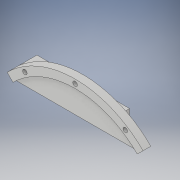
# Autodesk Inventor part: BearingGuard
Saved by Autodesk Inventor 2018 (Build 220112000, 112)
## iProperties
Created: 2019-02-07
Part Number: BearingGuard
Material: Generic
Document SubType Name: Modeling
Designer: anirudh
Density: 1 g/cm^3
Appearance: Default
Author: anirudh
Autodesk Inventor part; units mm, degrees
ref_plane "YZ Plane" through (0, 0, 0) normal (1, 0, 0) x (0, 1, 0)
ref_plane "XZ Plane" through (0, 0, 0) normal (0, 1, 0) x (-1, 0, 0)
ref_plane "XY Plane" through (0, 0, 0) normal (0, 0, 1) x (1, 0, 0)
sketch "Sketch1" plane through (0, 0, 0) normal (0, 0, 1) x (1, 0, 0)
  line L0 (0, 0) -> (101.6, 0)
  arc A0 (101.7181, 101.7181) -> (-0.1181, 101.7181) centre (50.8, 50.8) ccw
  arc A1 (106.4776, 106.4776) -> (-4.8776, 106.4776) centre (50.8, 50.8) ccw
  line L1 (0, 101.6) -> (-4.8776, 106.4776)
  line L2 (0, 101.6) -> (11.1798, 101.6) construction
  line L3 (101.6, 101.6) -> (106.4776, 106.4776)
  constraints: 8 end point, 4 point on circle, 2 centre point, 2 horizontal, 2 point on line, 1 coincident
extrude "Extrusion1" add sketch "Sketch1" along normal blind 2.54
sketch "Sketch2" plane through (0, 0, 0) normal (0, 0, -1) x (-1, 0, 0)
  line L0 (-101.7181, 101.7181) -> (0.1181, 101.7181)
  line L1 (-101.7181, 101.7181) -> (-106.4776, 106.4776) projected
  line L2 (-101.7181, 101.7181) -> (-106.4776, 106.4776)
  line L3 (4.8776, 106.4776) -> (0.1181, 101.7181) projected
  line L4 (0.1181, 101.7181) -> (4.8776, 106.4776)
  arc A0 (4.8776, 106.4776) -> (-106.4776, 106.4776) centre (-50.8, 50.8) ccw projected
  arc A1 (-106.4776, 106.4776) -> (-106.4776, 106.4776) centre (-50.8, 50.8) ccw
  point P0 (0, 0)
  constraints: 6 end point, 2 collinear, 1 horizontal, 4 other
extrude "Extrusion2" add sketch "Sketch2" along normal blind 3.81 contours L1 A0 L3 L0
sketch "Sketch8" plane through (0, 0, 2.54) normal (0, 0, 1) x (1, 0, 0)
  circle A0 centre (9.6434, 113.9463) radius 1.85
  circle A1 centre (50.8, 126.1745) radius 1.85
  circle A2 centre (91.9566, 113.9463) radius 1.85
  point P0 (0, 0)
  dimension "d32" = 3.7
  dimension "d33" = 3.7
  dimension "d34" = 3.7
  constraints: 3 centre point
  measures "d32" diameter of A0
  measures "d33" diameter of A1
  measures "d34" diameter of A2
extrude "Extrusion7" cut sketch "Sketch8" against normal blind 18.0594
sketch "Sketch9" plane through (0, 0, -3.81) normal (0, 0, -1) x (-1, 0, 0)
  line L0 (0.1181, 101.7181) -> (-71.0019, 101.7181)
  line L1 (0.1181, 101.7181) -> (4.8776, 106.4776) projected
  line L2 (0.1181, 101.7181) -> (4.8776, 106.4776)
  line L3 (4.8776, 106.4776) -> (-71.0019, 106.4776)
  line L4 (-71.0019, 106.4776) -> (-71.0019, 101.7181)
  point P0 (0, 0)
  dimension "d37" = 71.12
  constraints: 8 end point, 1 collinear, 1 horizontal
  measures "d37" distance of L0.start L0.end
extrude "Extrusion8" add sketch "Sketch9" along normal blind 18.0594
sketch "Sketch10" plane through (-4.8776, 106.4776, -3.81) normal (0, 1, 0) x (1, 0, 0)
  circle A0 centre (66.3545, 10.5594) radius 1.85
  circle A1 centre (19.05, 10.5594) radius 1.85
  circle A2 centre (42.7023, 10.5594) radius 1.85
  point P0 (4.8776, -3.81)
  point P1 (0, 18.0594)
  dimension "d44" = 3.7
  dimension "d45" = 3.7
  dimension "d46" = 3.7
  constraints: 3 centre point
  measures "d44" diameter of A0
  measures "d45" diameter of A1
  measures "d46" diameter of A2
extrude "Extrusion9" cut sketch "Sketch10" against normal blind 18.0594
fillet "Fillet3" radius 6.35 1 edges at (33.0622, 106.4776, -3.81)
fillet "Fillet4" radius 6.35 1 edges at (71.0019, 107.2728, -3.81)
body "Solid1"
